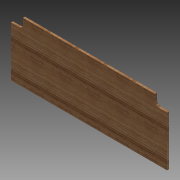
# Autodesk Inventor part: manipulator side pannel
Saved by Autodesk Inventor 2012 (Build 160160000, 160)
## iProperties
Created: 2013-09-02
Part Number: manipulator side pannel
Material: Default
Document SubType Name: Modeling
Designer: Bryce
Density: 1 g/cm^3
Author: Bryce
Autodesk Inventor part; units mm, degrees
ref_plane "YZ Plane" through (0, 0, 0) normal (1, 0, 0) x (0, 1, 0)
ref_plane "XZ Plane" through (0, 0, 0) normal (0, 1, 0) x (-1, 0, 0)
ref_plane "XY Plane" through (0, 0, 0) normal (0, 0, 1) x (1, 0, 0)
sketch "Sketch1" plane through (0, 0, 0) normal (0, 0, 1) x (1, 0, 0)
  line L0 (0, 0) -> (495.3, 0)
  line L1 (495.3, 0) -> (495.3, 158.75)
  line L2 (495.3, 190.5) -> (457.2, 190.5) construction
  line L3 (0, 190.5) -> (0, 158.75) construction
  arc A0 (25.4, 158.75) -> (38.1, 171.45) centre (25.4, 171.45) ccw
  arc A1 (457.2, 171.45) -> (469.9, 158.75) centre (469.9, 171.45) ccw
  line L4 (25.4, 158.75) -> (0, 158.75)
  line L5 (38.1, 171.45) -> (38.1, 190.5)
  line L6 (469.9, 158.75) -> (495.3, 158.75)
  line L7 (457.2, 171.45) -> (457.2, 190.5)
  line L8 (38.1, 190.5) -> (0, 190.5) construction
  line L9 (0, 158.75) -> (0, 0)
  line L10 (457.2, 190.5) -> (38.1, 190.5)
  line L11 (495.3, 158.75) -> (495.3, 190.5) construction
  dimension "d0" = 190.5
  dimension "d1" = 495.3
  dimension "d4" = 25.4
  dimension "d5" = 25.4
  dimension "d6" = 25.4
  dimension "d7" = 19.05
  dimension "d8" = 25.4
  dimension "d9" = 19.05
  constraints: 24 end point, 9 perpendicular, 7 parallel, 4 point on circle, 4 tangent, 2 centre point, 1 horizontal
  measures "d0" distance of L3.start L0.start
  measures "d1" distance of L2.start L3.start
  measures "d4" diameter of A0
  measures "d5" diameter of A1
  measures "d6" distance from line of L3 A0.centre
  measures "d7" distance from line of L2 A0.centre
  measures "d8" distance from line of L1 A1.centre
  measures "d9" distance from line of L2 A1.centre
extrude "Extrusion1" add sketch "Sketch1" against normal blind 6.35
equation "\"d5\" = d4"
equation "\"d8\" = d6"
equation "\"d9\" = d7"
body "Solid1"
